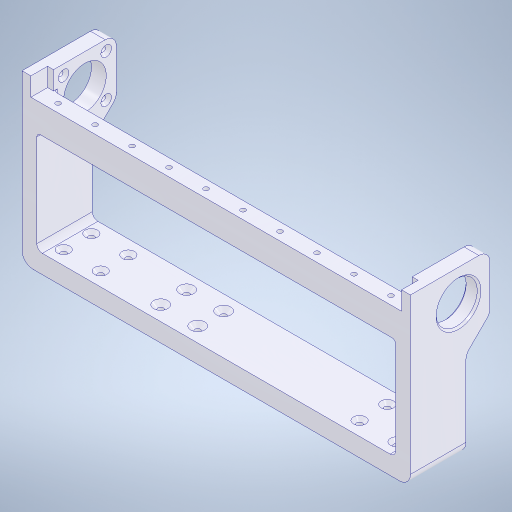
# Autodesk Inventor part: gantry_L
Saved by Autodesk Inventor 2024.1 (Build 281209000, 209)
## iProperties
Created: 2023-08-11
Part Number: gantry_L
Material: Generic
Document SubType Name: Modeling
Designer: l1534
Density: 1 g/cm^3
Appearance: Cool White
Author: l1534
Autodesk Inventor part; units mm, degrees
ref_plane "YZ Plane" through (0, 0, 0) normal (1, 0, 0) x (0, 1, 0)
ref_plane "XZ Plane" through (0, 0, 0) normal (0, 1, 0) x (-1, 0, 0)
ref_plane "XY Plane" through (0, 0, 0) normal (0, 0, 1) x (1, 0, 0)
sketch "Sketch1" plane through (0, 0, 0) normal (0, 0, 1) x (1, 0, 0)
  line L0 (-75.4115, 94.0727) -> (134.5885, 94.0727)
  line L1 (134.5885, 94.0727) -> (134.5885, 4.0727)
  line L2 (134.5885, 4.0727) -> (-75.4115, 4.0727)
  line L3 (-75.4115, 4.0727) -> (-75.4115, 94.0727)
  point P0 (0, 0)
  dimension "d0" = 210
  dimension "d1" = 90
  constraints: 8 end point, 2 parallel, 1 horizontal, 1 perpendicular
  measures "d0" distance of L0.start L0.end
  measures "d1" distance of L0.end L1.end
extrude "Extrusion1" add sketch "Sketch1" along normal blind 30
sketch "Sketch2" plane through (0, 0, 30) normal (0, 0, 1) x (1, 0, 0)
  line L0 (134.5885, 94.0727) -> (-75.4115, 94.0727) projected
  line L1 (-67.4115, 94.0727) -> (126.5885, 94.0727)
  line L2 (126.5885, 94.0727) -> (126.5885, 14.0727)
  line L3 (126.5885, 14.0727) -> (-67.4115, 14.0727)
  line L4 (-67.4115, 14.0727) -> (-67.4115, 94.0727)
  line L5 (-75.4115, 94.0727) -> (-75.4115, 4.0727) projected
  line L6 (134.5885, 4.0727) -> (134.5885, 94.0727) projected
  line L7 (-75.4115, 4.0727) -> (134.5885, 4.0727) projected
  point P0 (0, 0)
  dimension "d4" = 8
  dimension "d5" = 8
  dimension "d6" = 10
  constraints: 8 end point, 2 parallel, 1 horizontal, 1 perpendicular, 1 point on line
  measures "d4" distance between parallel lines of L5 L4
  measures "d5" distance between parallel lines of L6 L2
  measures "d6" distance between parallel lines of L7 L3
extrude "Extrusion2" cut sketch "Sketch2" against normal blind 30 contours L2 L3 L4 L0
sketch "Sketch3" plane through (-67.4115, 14.0727, 30) normal (0, 1, 0) x (1, 0, 0)
  circle A0 centre (7, 7.5) radius 1.5
  circle A1 centre (7, 22.5) radius 1.5
  circle A2 centre (27, 7.5) radius 1.5
  circle A3 centre (27, 22.5) radius 1.5
  circle A4 centre (187, 22.5) radius 1.5
  circle A5 centre (167, 7.5) radius 1.5
  circle A6 centre (187, 7.5) radius 1.5
  circle A7 centre (167, 22.5) radius 1.5
  line L0 (194, 0) -> (0, 0) projected
  line L1 (194, 30) -> (194, 0) projected
  point P0 (67.4115, 30)
  dimension "d9" = 3
  dimension "d10" = 3
  dimension "d11" = 3
  dimension "d12" = 3
  dimension "d13" = 3
  dimension "d14" = 3
  dimension "d15" = 3
  dimension "d16" = 3
  dimension "d18" = 7.5
  dimension "d19" = 7.5
  dimension "d20" = 7.5
  dimension "d21" = 7.5
  dimension "d22" = 20
  dimension "d23" = 20
  dimension "d24" = 7
  dimension "d25" = 20
  dimension "d26" = 20
  dimension "d27" = 7
  dimension "d28" = 15
  dimension "d29" = 15
  dimension "d30" = 15
  dimension "d31" = 15
  dimension "d33" = 140
  dimension "d34" = 140
  constraints: 8 centre point
  measures "d9" diameter of A0
  measures "d10" diameter of A1
  measures "d11" diameter of A2
  measures "d12" diameter of A3
  measures "d13" diameter of A6
  measures "d14" diameter of A7
  measures "d15" diameter of A5
  measures "d16" diameter of A4
  measures "d18" distance from line of L0 A6.centre
  measures "d19" distance from line of L0 A2.centre
  measures "d20" distance from line of L0 A0.centre
  measures "d21" distance from line of L0 A5.centre
  measures "d22" distance of A2.centre A0.centre
  measures "d23" distance of A3.centre A1.centre
  measures "d24" distance from line of L1 A6.centre
  measures "d25" distance of A6.centre A5.centre
  measures "d26" distance of A7.centre A4.centre
  measures "d27" distance from line of L1 A4.centre
  measures "d28" distance of A4.centre A6.centre
  measures "d29" distance of A5.centre A7.centre
  measures "d30" distance of A2.centre A3.centre
  measures "d31" distance of A0.centre A1.centre
  measures "d33" distance of A5.centre A2.centre
  measures "d34" distance of A7.centre A3.centre
extrude "Extrusion3" cut sketch "Sketch3" against normal blind 30
chamfer "Chamfer1" distance 1.8 angle 45 8 edges at (-61.9115, 14.0727, 7.5) (-61.9115, 14.0727, 22.5) (-41.9115, 14.0727, 22.5) (-41.9115, 14.0727, 7.5) (118.0885, 14.0727, 7.5) (118.0885, 14.0727, 22.5) (98.0885, 14.0727, 22.5) (98.0885, 14.0727, 7.5)
sketch "Sketch9" plane through (0, 0, 0) normal (0, 0, -1) x (-1, 0, 0)
  line L0 (-134.5885, 94.0727) -> (-126.5885, 94.0727) projected
  line L1 (-134.5885, 94.0727) -> (-126.5885, 94.0727)
  line L2 (-126.5885, 94.0727) -> (-126.5885, 64.0727)
  line L3 (-126.5885, 64.0727) -> (-134.5885, 64.0727)
  line L4 (-134.5885, 64.0727) -> (-134.5885, 94.0727)
  line L5 (67.4115, 94.0727) -> (75.4115, 94.0727) projected
  line L6 (67.4115, 94.0727) -> (67.4115, 14.0727) projected
  line L7 (75.4115, 94.0727) -> (67.4115, 94.0727)
  line L8 (67.4115, 94.0727) -> (67.4115, 64.0727)
  line L9 (67.4115, 64.0727) -> (75.4115, 64.0727)
  line L10 (75.4115, 64.0727) -> (75.4115, 94.0727)
  point P0 (0, 0)
  point P1 (71.4115, 94.0727)
  point P2 (71.4115, 64.0727)
  dimension "d74" = 30
  dimension "d75" = 30
  dimension "d90" = 8
  constraints: 16 end point, 4 parallel, 2 horizontal, 2 midpoint, 2 perpendicular, 1 point on line
  measures "d74" distance of L1.end L2.end
  measures "d75" distance of point (71.411, 94.073) point (71.411, 64.073)
  measures "d90" distance between parallel lines of L4 L2
extrude "Extrusion9" add sketch "Sketch9" along normal blind 13
chamfer "Chamfer4" distance 13 angle 45 2 edges at (130.5885, 64.0727, 0) (-71.4115, 64.0727, 0)
sketch "Sketch12" plane through (-67.4115, 14.0727, 30) normal (1, 0, 0) x (0, 0, -1)
  line L0 (0, 0) -> (0, 80) projected
  line L1 (0, 70) -> (9, 70)
  line L2 (9, 70) -> (9, 55)
  line L3 (9, 55) -> (0, 55)
  line L4 (0, 55) -> (0, 70)
  line L5 (0, 80) -> (43, 80) projected
  point P0 (30, -14.0727)
  point P1 (0, 55)
  dimension "d97" = 9
  dimension "d98" = 15
  dimension "d99" = 10
  constraints: 8 end point, 2 parallel, 1 horizontal, 1 perpendicular, 1 point on line
  measures "d97" distance of L1.start L1.end
  measures "d98" distance of L1.end L2.end
  measures "d99" distance between parallel lines of L5 L1
extrude "Extrusion12" add sketch "Sketch12" along normal blind 194
sketch "Sketch13" plane through (-75.4115, 4.0727, 30) normal (-1, 0, 0) x (0, 0, 1)
  circle A0 centre (-26, 73) radius 11.5
  line L0 (-43, 90) -> (0, 90) projected
  line L1 (-43, 60) -> (-43, 90) projected
  circle A1 centre (-37.5, 84.5) radius 1.25
  circle A2 centre (-14.5, 84.5) radius 1.25
  circle A3 centre (-14.5, 61.5) radius 1.25
  circle A4 centre (-37.5, 61.5) radius 1.25
  point P0 (-30, -4.0727)
  dimension "d102" = 23
  dimension "d103" = 17
  dimension "d104" = 17
  dimension "d128" = 2.5
  dimension "d129" = 2.5
  dimension "d130" = 2.5
  dimension "d131" = 2.5
  dimension "d132" = 11.5
  dimension "d133" = 11.5
  dimension "d134" = 11.5
  dimension "d135" = 11.5
  dimension "d136" = 11.5
  dimension "d137" = 11.5
  dimension "d138" = 11.5
  dimension "d139" = 11.5
  constraints: 5 centre point
  measures "d102" diameter of A0
  measures "d103" distance from line of L0 A0.centre
  measures "d104" distance from line of L1 A0.centre
  measures "d128" diameter of A1
  measures "d129" diameter of A2
  measures "d130" diameter of A3
  measures "d131" diameter of A4
  measures "d132" horizontal distance of A0.centre A4.centre
  measures "d133" horizontal distance of A0.centre A4.centre
  measures "d134" horizontal distance of A0.centre A3.centre
  measures "d135" horizontal distance of A0.centre A3.centre
  measures "d136" horizontal distance of A0.centre A2.centre
  measures "d137" horizontal distance of A0.centre A2.centre
  measures "d138" horizontal distance of A0.centre A1.centre
  measures "d139" horizontal distance of A0.centre A1.centre
extrude "Extrusion13" cut sketch "Sketch13" against normal blind 202
fillet "Fillet3" radius 2 4 edges at (-67.4115, 76.5727, 21) (-67.4115, 69.0727, 25.5) (126.5885, 76.5727, 21) (126.5885, 69.0727, 25.5)
sketch "Sketch14" plane through (-75.4115, 94.0727, 30) normal (0, 1, 0) x (1, 0, 0)
  line L0 (8, 0) -> (0, 0) projected
  line L1 (4.8, 0) -> (205.2, 0)
  line L2 (205.2, 0) -> (205.2, 9)
  line L3 (205.2, 9) -> (4.8, 9)
  line L4 (4.8, 9) -> (4.8, 0)
  line L5 (202, 43) -> (202, 0) projected
  line L6 (8, 0) -> (8, 43) projected
  point P0 (75.4115, 30)
  point P1 (202, 9)
  point P2 (8, 9)
  dimension "d108" = 9
  dimension "d109" = 3.2
  dimension "d110" = 3.2
  constraints: 8 end point, 2 parallel, 1 horizontal, 1 perpendicular, 1 point on line
  measures "d108" distance of L1.end L2.end
  measures "d109" distance between parallel lines of L5 L2
  measures "d110" distance between parallel lines of L6 L4
extrude "Extrusion14" cut sketch "Sketch14" against normal blind 10 contours L0 L4 L3 L6 | L5 L3 L2 L1
sketch "Sketch15" plane through (-65.4115, 84.0727, 21) normal (0, 1, 0) x (1, 0, 0)
  circle A0 centre (5, -4.5) radius 1.3
  line L0 (-5.2, -9) -> (-5.2, 0) projected
  line L1 (195.2, -9) -> (-5.2, -9) projected
  circle A1 centre (25, -4.5) radius 1.3
  circle A2 centre (45, -4.5) radius 1.3
  circle A3 centre (65, -4.5) radius 1.3
  circle A4 centre (85, -4.5) radius 1.3
  circle A5 centre (105, -4.5) radius 1.3
  circle A6 centre (125, -4.5) radius 1.3
  circle A7 centre (145, -4.5) radius 1.3
  circle A8 centre (165, -4.5) radius 1.3
  circle A9 centre (185, -4.5) radius 1.3
  point P0 (65.4115, 21)
  dimension "d116" = 10.2
  dimension "d117" = 4.5
  dimension "d120" = 20
  dimension "d127" = 2.6
  constraints: 10 centre point, 1 horizontal, 18 other
  measures "d116" distance from line of L0 A0.centre
  measures "d117" distance from line of L1 A0.centre
  measures "d120" distance of A0.centre A1.centre
  measures "d127" diameter of A0
extrude "Extrusion15" cut sketch "Sketch15" against normal blind 15
chamfer "Chamfer9" distance 1.6 angle 45 4 edges at (-67.4115, 88.5727, 14.25) (-67.4115, 88.5727, -8.75) (-67.4115, 65.5727, 14.25) (-67.4115, 65.5727, -8.75)
fillet "Fillet4" radius 3 2 edges at (126.5885, 14.0727, 15) (-67.4115, 14.0727, 15)
fillet "Fillet5" radius 6 2 edges at (134.5885, 4.0727, 15) (-75.4115, 4.0727, 15)
fillet "Fillet6" radius 6 12 edges at (130.5885, 51.0728, 0) (-71.4115, 51.0728, 0) (-75.4115, 64.0727, -13) (-67.4115, 64.0727, -13) (-71.4115, 64.0727, -12.9999) (-71.4115, 64.0727, -13) (134.5885, 64.0727, -13) (126.5885, 64.0727, -13) (130.5885, 64.0727, -12.9999) (130.5885, 64.0727, -13) (130.5885, 94.0727, -13) (-71.4115, 94.0727, -13)
sketch "Sketch17" plane through (-64.4115, 14.0727, 30) normal (0, 1, 0) x (1, 0, 0)
  circle A0 centre (56, 22) radius 1.5
  circle A1 centre (56, 8) radius 1.5
  circle A2 centre (76, 8) radius 1.5
  circle A3 centre (76, 22) radius 1.5
  line L0 (0, 30) -> (188, 30) projected
  line L1 (188, 0) -> (0, 0) projected
  line L2 (-3, 30) -> (-3, 0) projected
  point P0 (64.4115, 30)
  dimension "d155" = 3
  dimension "d156" = 3
  dimension "d157" = 3
  dimension "d158" = 3
  dimension "d159" = 8
  dimension "d160" = 8
  dimension "d161" = 8
  dimension "d162" = 8
  dimension "d163" = 20
  dimension "d164" = 20
  dimension "d165" = 59
  dimension "d166" = 59
  constraints: 4 centre point
  measures "d155" diameter of A1
  measures "d156" diameter of A0
  measures "d157" diameter of A2
  measures "d158" diameter of A3
  measures "d159" distance from line of L0 A0.centre
  measures "d160" distance from line of L1 A1.centre
  measures "d161" distance from line of L0 A3.centre
  measures "d162" distance from line of L1 A2.centre
  measures "d163" distance of A3.centre A0.centre
  measures "d164" distance of A2.centre A1.centre
  measures "d165" distance from line of L2 A0.centre
  measures "d166" distance from line of L2 A1.centre
extrude "Extrusion17" cut sketch "Sketch17" against normal blind 10
chamfer "Chamfer10" distance 2.3 angle 45 4 edges at (10.0885, 14.0727, 22) (-9.9115, 14.0727, 22) (-9.9115, 14.0727, 8) (10.0885, 14.0727, 8)
sketch "Sketch18" plane through (134.5885, 10.0727, 30) normal (1, 0, 0) x (0, 0, -1)
  circle A0 centre (26, 67) radius 11.5 projected
  circle A1 centre (26, 67) radius 11.1
  point P0 (30, -10.0727)
  dimension "d172" = 22.2
  constraints: 1 centre point, 1 coincident
  measures "d172" diameter of A1
extrude "Extrusion18" cut sketch "Sketch18" against normal up to surface (8 mm away) contours A1
chamfer "Chamfer11" distance 1 angle 45 2 edges at (126.5885, 77.0727, 15.1) (134.5885, 77.0727, 15.1)
equation "\"d20\" = d19"
equation "\"d21\" = d18"
equation "\"d23\" = d22"
equation "\"d26\" = d25"
equation "\"d27\" = d24"
equation "\"d29\" = d28"
equation "\"d30\" = d29"
equation "\"d31\" = d30"
equation "\"d34\" = d33"
body "Solid1"
